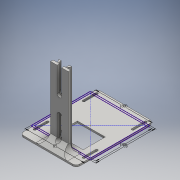
# Autodesk Inventor part: Line sensor hold 1
Saved by Autodesk Inventor 2016 (Build 200138000, 138)
## iProperties
Created: 2018-02-27
Part Number: Line sensor hold 1
Material: Generic
Document SubType Name: Modeling
Designer: ALIREZA
Density: 1 g/cm^3
Appearance: Default
Author: ALIREZA
Autodesk Inventor part; units mm, degrees
ref_plane "YZ Plane" through (0, 0, 0) normal (1, 0, 0) x (0, 1, 0)
ref_plane "XZ Plane" through (0, 0, 0) normal (0, 1, 0) x (-1, 0, 0)
ref_plane "XY Plane" through (0, 0, 0) normal (0, 0, 1) x (1, 0, 0)
sketch "Sketch1" plane through (0, 0, 0) normal (0, 0, 1) x (1, 0, 0)
  line L0 (-40, -40) -> (40, -40)
  line L1 (40, -40) -> (40, 40)
  line L2 (40, 40) -> (-40, 40)
  line L3 (-40, 40) -> (-40, -40)
  line L4 (-40, -40) -> (40, 40) construction
  line L5 (40, -40) -> (-40, 40) construction
  line L6 (-40, -40) -> (-35, -40)
  line L7 (-40, -35) -> (-40, -40)
  circle A0 centre (-35, -35) radius 1.6
  circle A1 centre (-35, 35) radius 1.6
  line L8 (0, 0) -> (0, 27.2708) construction
  circle A2 centre (35, -35) radius 1.6
  circle A3 centre (35, 35) radius 1.6
  dimension "d0" = 80
  dimension "d1" = 80
  dimension "d4" = 3.2
  constraints: 18 end point, 4 centre point, 2 horizontal, 2 midpoint, 2 parallel, 2 symmetric about line, 1 perpendicular, 1 vertical, 2 other
  measures "d0" distance of L2.end L1.end
  measures "d1" distance of L1.end L0.end
  measures "d4" diameter of A0
extrude "Extrusion1" add sketch "Sketch1" along normal blind 2.5
sketch "Sketch2" plane through (0, 0, 2.5) normal (0, 0, 1) x (1, 0, 0)
  line L0 (40, -40) -> (40, 40) projected
  line L1 (40, -40) -> (5, -40) construction
  line L2 (5, -40) -> (5, -18.488) construction
  line L3 (-14.05, -13.283) -> (24.05, -13.283)
  line L4 (24.05, -13.283) -> (24.05, -23.693)
  line L5 (24.05, -23.693) -> (-14.05, -23.693)
  line L6 (-14.05, -23.693) -> (-14.05, -13.283)
  line L7 (-14.05, -13.283) -> (24.05, -23.693) construction
  line L8 (24.05, -13.283) -> (-14.05, -23.693) construction
  line L9 (5, -18.488) -> (5, -48.988) construction
  line L10 (5, -48.988) -> (17.5, -48.988)
  line L11 (17.5, -48.988) -> (-7.5, -48.988)
  line L12 (-7.5, -48.988) -> (-7.5, -45.488)
  line L13 (-7.5, -45.488) -> (17.5, -45.488) construction
  line L14 (17.5, -45.488) -> (17.5, -48.988)
  line L15 (-7.5, -48.988) -> (-7.5, -45.488)
  line L16 (-7.5, -40.488) -> (17.5, -40.488) construction
  line L17 (5, -45.488) -> (-7.5, -45.488) construction
  line L18 (5, -45.488) -> (-1.25, -45.488) construction
  line L19 (-7.5, -40.488) -> (-4.375, -40.488) construction
  line L20 (-4.375, -40.488) -> (-1.25, -45.488)
  line L21 (14.375, -40.488) -> (11.25, -45.488)
  line L22 (-1.25, -45.488) -> (-7.5, -45.488)
  line L23 (11.25, -45.488) -> (17.5, -45.488)
  line L24 (17.5, -48.988) -> (17.5, -45.488)
  line L25 (17.5, -48.988) -> (17.5, -45.488)
  ellipse E0 centre (5, -40.488) end of major axis (11.25, -40.488) minor radius 2.0521 (-1.25, -40.488) -> (11.25, -40.488) ccw
  line L26 (-4.375, -40.488) -> (-1.25, -40.488)
  line L27 (11.25, -40.488) -> (14.375, -40.488)
  circle A0 centre (35, -35) radius 1.6 projected
  circle A1 centre (35, 35) radius 1.6 projected
  circle A2 centre (-35, 35) radius 1.6 projected
  circle A3 centre (-35, -35) radius 1.6 projected
  line L28 (40, 40) -> (-40, 40) projected
  line L29 (40, 40) -> (40, -60) projected
  line L30 (-40, 40) -> (-40, -60) projected
  line L31 (40, -60) -> (-40, -60) projected
  circle A4 centre (35, -35) radius 1.6 projected
  circle A5 centre (35, 35) radius 1.6 projected
  circle A6 centre (-35, 35) radius 1.6 projected
  circle A7 centre (-35, -35) radius 1.6 projected
  line L32 (-40, -40) -> (-40, 40) projected
  line L33 (-40, 40) -> (40, 40) projected
  line L34 (40, 40) -> (40, -40) projected
  line L35 (40, -40) -> (-40, -40) projected
  point P0 (0, 0)
  dimension "d8" = 35
  dimension "d10" = 38.1
  dimension "d11" = 10.41
  dimension "d12" = 30.5
  dimension "d15" = 12.5
  dimension "d16" = 25
  dimension "d17" = 3.5
  dimension "d18" = 8.5
  dimension "d20" = 6.25
  dimension "d21" = 3.125
  constraints: 54 end point, 7 collinear, 4 midpoint, 3 perpendicular, 3 point on line, 3 vertical, 2 horizontal, 2 parallel, 2 symmetric about line, 4 other
  measures "d8" distance of L0.start L1.end
  measures "d10" distance of L4.end L5.end
  measures "d11" distance of L3.end L4.end
  measures "d12" distance of L2.end L9.end
  measures "d15" distance of L9.end L10.end
  measures "d16" distance of L10.end L11.end
  measures "d17" distance of L12.end L11.end
  measures "d18" distance of L11.end L16.start
  measures "d20" distance of L17.start L18.end
  measures "d21" distance of L16.start L19.end
sketch "Sketch3" plane through (0, 0, 2.5) normal (0, 0, 1) x (1, 0, 0)
  point P0 (0, 0)
sketch "Sketch4" plane through (0, 0, 2.5) normal (0, 0, 1) x (1, 0, 0)
  line L0 (-40, -40) -> (40, -40) projected
  line L1 (-40, -40) -> (40, -40)
  line L2 (40, -40) -> (40, -60)
  line L3 (40, -60) -> (-40, -60)
  line L4 (-40, -60) -> (-40, -40)
  point P0 (0, 0)
  dimension "d22" = 20
  constraints: 8 end point, 2 parallel, 1 horizontal, 1 perpendicular
  measures "d22" distance of L1.end L2.end
extrude "Extrusion3" add sketch "Sketch4" against normal blind 2.5
extrude "Extrusion4" add sketch "Sketch2" along normal blind 100 contours L11 L12 L22 L20 L26 E0 L27 L21 L23 L14 L10
sketch "Sketch5" plane through (0, 0, 2.5) normal (0, 0, 1) x (1, 0, 0)
  point P0 (0, 0)
sketch "Sketch6" plane through (0, 0, 2.5) normal (0, 0, 1) x (1, 0, 0)
  line L0 (5, -40) -> (5, -18.488) construction
  line L1 (-14.05, -13.283) -> (24.05, -13.283)
  line L2 (24.05, -13.283) -> (24.05, -23.693)
  line L3 (24.05, -23.693) -> (-14.05, -23.693)
  line L4 (-14.05, -23.693) -> (-14.05, -13.283)
  line L5 (-14.05, -13.283) -> (24.05, -23.693) construction
  line L6 (24.05, -13.283) -> (-14.05, -23.693) construction
  line L7 (5, -18.488) -> (5, -48.988) construction
  point P0 (0, 0)
  dimension "d27" = 38.1
  dimension "d28" = 10.41
  dimension "d29" = 30.5
  constraints: 16 end point, 2 midpoint, 2 parallel, 1 horizontal, 1 perpendicular, 1 point on line, 1 vertical
  measures "d27" distance of L3.start L4.start
  measures "d28" distance of L1.end L3.start
  measures "d29" distance of L0.end L7.end
extrude "Extrusion5" cut sketch "Sketch6" against normal blind 50
sketch "Sketch7" plane through (11.25, -40.488, 2.5) normal (0, 1, 0) x (1, 0, 0)
  line L0 (0, -100) -> (-12.5, -100) projected
  line L1 (-6.25, -100) -> (-6.25, -85) construction
  line L2 (-6.25, -65) -> (-6.25, -105) construction
  line L3 (-9.55, -65) -> (-9.55, -105)
  line L4 (-2.95, -105) -> (-2.95, -65)
  arc A0 (-2.95, -65) -> (-9.55, -65) centre (-6.25, -65) ccw
  arc A1 (-9.55, -105) -> (-2.95, -105) centre (-6.25, -105) ccw
  line L5 (-6.25, -10) -> (-6.25, -40) construction
  line L6 (-9.5, -10) -> (-9.5, -40)
  line L7 (-3, -40) -> (-3, -10)
  arc A2 (-3, -10) -> (-9.5, -10) centre (-6.25, -10) ccw
  arc A3 (-9.5, -40) -> (-3, -40) centre (-6.25, -40) ccw
  point P0 (-11.25, 2.5)
  point P1 (-6.25, -25)
  dimension "d32" = 15
  dimension "d33" = 20
  dimension "d34" = 6.6
  dimension "d35" = 15
  dimension "d36" = 6.5
  constraints: 18 end point, 8 point on circle, 8 tangent, 4 centre point, 3 midpoint, 3 vertical, 2 parallel
  measures "d32" distance of L1.start L1.end
  measures "d33" distance of L1.end L2.end
  measures "d34" diameter of A1
  measures "d35" distance of point (-6.25, -25) L5.end
  measures "d36" diameter of A3
extrude "Extrusion6" cut sketch "Sketch7" against normal blind 50
sketch "Sketch8" plane through (11.25, -40.488, 2.5) normal (0, 1, 0) x (1, 0, 0)
  line L0 (-9.55, -100) -> (-9.55, -65) projected
  arc A0 (-3, -10) -> (-9.5, -10) centre (-6.25, -10) ccw projected
  arc A1 (-9.5, -40) -> (-3, -40) centre (-6.25, -40) ccw projected
  line L1 (-6.25, -10) -> (-6.25, -40) construction
  line L2 (-6.25, -65) -> (-6.25, -109.4908) construction
  line L3 (-6.25, -10) -> (-6.25, -40) construction
  line L4 (-3, -40) -> (-3, -10) projected
  line L5 (-11.75, -10) -> (-11.75, -40)
  line L6 (-0.75, -40) -> (-0.75, -10)
  arc A2 (-0.75, -10) -> (-11.75, -10) centre (-6.25, -10) ccw
  arc A3 (-11.75, -40) -> (-0.75, -40) centre (-6.25, -40) ccw
  line L7 (-6.25, -65) -> (-6.25, -109.4908) construction
  line L8 (-11.75, -65) -> (-11.75, -109.4908)
  line L9 (-0.75, -109.4908) -> (-0.75, -65)
  arc A4 (-0.75, -65) -> (-11.75, -65) centre (-6.25, -65) ccw
  arc A5 (-11.75, -109.4908) -> (-0.75, -109.4908) centre (-6.25, -109.4908) ccw
  point P0 (-11.25, 2.5)
  point P1 (-6.25, -25)
  point P2 (-6.25, -87.2454)
  dimension "d39" = 11
  dimension "d40" = 11
  constraints: 20 end point, 8 point on circle, 8 tangent, 4 centre point, 4 equal length, 2 midpoint, 2 vertical, 1 horizontal alignment
  measures "d39" diameter of A3
  measures "d40" diameter of A5
extrude "Extrusion7" cut sketch "Sketch8" against normal blind 5
fillet "Fillet1" radius 10 1 edges at (17.5, -47.238, 2.5)
fillet "Fillet2" radius 10 1 edges at (-7.5, -47.238, 2.5)
fillet "Fillet4" radius 5 2 edges at (22.5, -45.488, 2.5) (14.375, -45.488, 2.5)
fillet "Fillet5" radius 5 2 edges at (-4.375, -45.488, 2.5) (-12.5, -45.488, 2.5)
chamfer "Chamfer1" distance 11 angle 45 3 edges at (-12.5, -48.988, 2.5) (5, -48.988, 2.5) (22.5, -48.988, 2.5)
sketch "Sketch9" plane through (0, 0, 2.5) normal (0, 0, 1) x (1, 0, 0)
  line L0 (-14.05, -13.283) -> (24.05, -13.283) projected
  line L1 (24.05, -13.283) -> (24.05, -23.693) projected
  line L2 (24.05, -23.693) -> (-14.05, -23.693) projected
  line L3 (-14.05, -23.693) -> (-14.05, -13.283) projected
  line L4 (24.85, -12.483) -> (-14.85, -12.483)
  line L5 (-14.85, -12.483) -> (-14.85, -24.493)
  line L6 (-14.85, -24.493) -> (24.85, -24.493)
  line L7 (24.85, -24.493) -> (24.85, -12.483)
  line L8 (5, -19.774) -> (5, -24.493)
  line L9 (-7.5, -48.988) -> (1.7, -48.988) projected
  line L10 (0, -48.988) -> (-26, -48.988)
  line L11 (24.85, -35) -> (-14.85, -35)
  line L12 (-14.85, -35) -> (-14.85, -3.417)
  line L13 (-14.85, -3.417) -> (24.85, -3.417)
  line L14 (24.85, -3.417) -> (24.85, -35)
  point P0 (0, 0)
  dimension "d51" = 0.8
  dimension "d52" = 26
  constraints: 20 end point, 2 parallel, 1 collinear, 1 horizontal, 1 midpoint, 1 perpendicular, 1 point on line, 3 other
  measures "d51" distance between parallel lines of L0 L4
  measures "d52" distance of L10.start L10.end
extrude "Extrusion8" cut sketch "Sketch9" against normal blind 14 contours L0 L1 L2 L3 | L7 L6 L5 L4 | L4 L12 L13 L14 | L14 L11 L12 L6
sketch "Sketch10" plane through (0, 0, 2.5) normal (0, 0, 1) x (1, 0, 0)
  line L0 (-42.5, 42.5) -> (42.5, 42.5)
  line L1 (42.5, 42.5) -> (42.5, -42.5)
  line L2 (42.5, -42.5) -> (-42.5, -42.5)
  line L3 (-42.5, -42.5) -> (-42.5, 42.5)
  line L4 (-42.5, 42.5) -> (42.5, -42.5) construction
  line L5 (42.5, 42.5) -> (-42.5, -42.5) construction
  line L6 (-40, -40) -> (40, -40)
  line L7 (40, -40) -> (40, 40)
  line L8 (40, 40) -> (-40, 40)
  line L9 (-40, 40) -> (-40, -40)
  line L10 (-40, -40) -> (40, 40) construction
  line L11 (40, -40) -> (-40, 40) construction
  point P0 (0, 0)
  dimension "d56" = 85
  dimension "d57" = 85
  dimension "d58" = 80
  dimension "d59" = 80
  constraints: 24 end point, 4 midpoint, 4 parallel, 2 horizontal, 2 perpendicular
  measures "d56" distance of L1.end L2.end
  measures "d57" distance of L0.end L1.end
  measures "d58" distance of L8.end L7.end
  measures "d59" distance of L7.end L6.end
sketch "Sketch11" plane through (0, 0, 2.5) normal (0, 0, 1) x (1, 0, 0)
  line L0 (40, 40) -> (-40, 40) projected
  line L1 (-40, 40) -> (40, 40)
  line L2 (40, 40) -> (40, 50)
  line L3 (40, 50) -> (-40, 50)
  line L4 (-40, 50) -> (-40, 40)
  point P0 (0, 0)
  dimension "d60" = 10
  constraints: 8 end point, 2 parallel, 1 horizontal, 1 perpendicular
  measures "d60" distance of L2.end L1.end
extrude "Extrusion9" add sketch "Sketch11" against normal up to surface (2.5 mm away)
sketch "Sketch12" plane through (0, 0, 2.5) normal (0, 0, 1) x (1, 0, 0)
  line L0 (-35, 44.2357) -> (-35, 25.7643) construction
  circle A0 centre (-35, 35) radius 1.6 projected
  line L1 (-36.6, 44.2357) -> (-36.6, 25.7643)
  line L2 (-33.4, 25.7643) -> (-33.4, 44.2357)
  arc A1 (-33.4, 44.2357) -> (-36.6, 44.2357) centre (-35, 44.2357) ccw
  arc A2 (-36.6, 25.7643) -> (-33.4, 25.7643) centre (-35, 25.7643) ccw
  line L3 (0, 0) -> (-14.7609, 0) construction
  line L4 (-14.7609, 0) -> (0, 0)
  line L5 (0, 0) -> (0, 10.1253) construction
  line L6 (-36.6, -44.2357) -> (-36.6, -25.7643)
  line L7 (-33.4, -25.7643) -> (-33.4, -44.2357)
  arc A3 (-36.6, -44.2357) -> (-33.4, -44.2357) centre (-35, -44.2357) ccw
  arc A4 (-33.4, -25.7643) -> (-36.6, -25.7643) centre (-35, -25.7643) ccw
  line L8 (0, 0) -> (0, -10.1253) construction
  line L9 (36.6, 44.2357) -> (36.6, 25.7643)
  line L10 (33.4, 25.7643) -> (33.4, 44.2357)
  arc A5 (36.6, 44.2357) -> (33.4, 44.2357) centre (35, 44.2357) ccw
  arc A6 (33.4, 25.7643) -> (36.6, 25.7643) centre (35, 25.7643) ccw
  line L11 (33.4, -25.7643) -> (33.4, -44.2357)
  arc A7 (33.4, -44.2357) -> (36.6, -44.2357) centre (35, -44.2357) ccw
  line L12 (36.6, -44.2357) -> (36.6, -25.7643)
  arc A8 (36.6, -25.7643) -> (33.4, -25.7643) centre (35, -25.7643) ccw
  constraints: 28 end point, 19 symmetric about line, 16 point on circle, 8 centre point, 4 tangent, 2 equal length, 2 vertical, 1 horizontal, 1 midpoint, 6 other
extrude "Extrusion10" cut sketch "Sketch12" against normal blind 14 contours L2 A2 L1 A0 | A0 L1 A1 L2 | L6 A4 L7 A3 | L9 A6 L10 A5 | A8 L12 A7 L11
fillet "Fillet6" radius 5 1 edges at (40, 50, 1.25)
fillet "Fillet7" radius 5 1 edges at (-40, 50, 1.25)
fillet "Fillet8" radius 5 1 edges at (40, -60, 1.25)
fillet "Fillet9" radius 5 1 edges at (-40, -60, 1.25)
body "Solid1"
